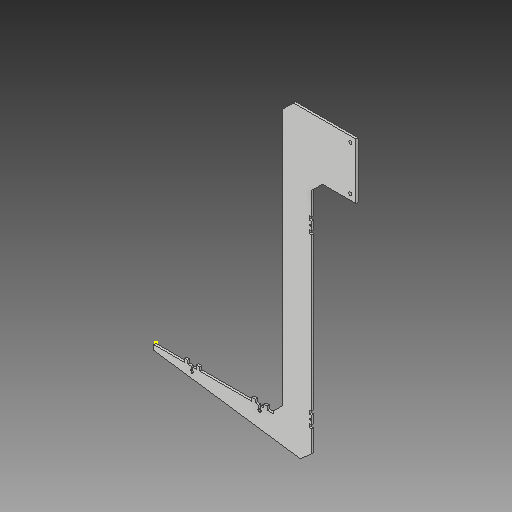
# Autodesk Inventor part: Z stage_side
Saved by Autodesk Inventor 2019 (Build 230136000, 136)
## iProperties
Created: 2020-03-07
Part Number: Z stage_side
Material: Generic
Document SubType Name: Modeling
Designer: Vijay
Density: 1 g/cm^3
Appearance: Default
Author: Vijay
Autodesk Inventor part; units mm, degrees
ref_plane "YZ Plane" through (0, 0, 0) normal (1, 0, 0) x (0, 1, 0)
ref_plane "XZ Plane" through (0, 0, 0) normal (0, 1, 0) x (-1, 0, 0)
ref_plane "XY Plane" through (0, 0, 0) normal (0, 0, 1) x (1, 0, 0)
sketch "Sketch1" plane through (0, 0, 0) normal (0, 0, 1) x (1, 0, 0)
  line L0 (230, 0) -> (0, 0) projected
  line L1 (0, 0) -> (0, -8.9243)
  line L2 (0, -8.9243) -> (282.1829, -48.5825)
  line L3 (282.1829, -48.5825) -> (282.1829, 400)
  line L4 (230, 0) -> (230, 500)
  line L5 (282.1829, 400) -> (362.1829, 400)
  line L6 (230, 500) -> (362.1829, 500)
  line L7 (362.1829, 500) -> (362.1829, 400)
  dimension "d0" = 400
  dimension "d1" = 8
  dimension "d10" = 80
  dimension "d11" = 100
  constraints: 14 end point, 2 horizontal, 2 vertical, 1 parallel, 1 perpendicular
  measures "d0" distance between parallel lines of L0 L5
  measures "d1" angle of L2 L0
  measures "d10" distance between parallel lines of L7 L3
  measures "d11" distance of L6.end L5.end
extrude "Extrusion1" add sketch "Sketch1" along normal blind 4
chamfer "Chamfer1" distance 20 angle 45 2 edges at (230, 500, 2) (282.1829, 400, 2)
chamfer "Chamfer2" distance 20 angle 45 2 edges at (230, 0, 2) (282.1829, -48.5825, 2)
sketch "Sketch2" plane through (0, 0, 0) normal (0, 0, -1) x (-1, 0, 0)
  point P0 (0, 0)
sketch "Sketch3" plane through (0, 0, 0) normal (0, 0, -1) x (-1, 0, 0)
  point P0 (0, 0)
sketch "Sketch4" plane through (0, 0, 0) normal (0, 0, -1) x (-1, 0, 0)
  point P0 (0, 0)
sketch "Sketch5" plane through (0, 0, 0) normal (0, 0, -1) x (-1, 0, 0)
  line L0 (-278.1829, 10.465) -> (-278.1829, 16.465) construction
  line L1 (-282.1829, 16.465) -> (-278.1829, 16.465) construction
  line L2 (-282.1829, 10.465) -> (-282.1829, 16.465) construction
  line L3 (-282.1829, 10.465) -> (-278.1829, 10.465) construction
  line L4 (-278.1829, 31.665) -> (-278.1829, 37.665) construction
  line L5 (-282.1829, 37.665) -> (-278.1829, 37.665) construction
  line L6 (-282.1829, 31.665) -> (-282.1829, 37.665) construction
  line L7 (-282.1829, 31.665) -> (-278.1829, 31.665) construction
  line L8 (-278.1829, 332.8339) -> (-278.1829, 338.8339) construction
  line L9 (-282.1829, 338.8339) -> (-278.1829, 338.8339) construction
  line L10 (-282.1829, 332.8339) -> (-282.1829, 338.8339) construction
  line L11 (-282.1829, 332.8339) -> (-278.1829, 332.8339) construction
  line L12 (-278.1829, 311.6339) -> (-278.1829, 317.6339) construction
  line L13 (-282.1829, 317.6339) -> (-278.1829, 317.6339) construction
  line L14 (-282.1829, 311.6339) -> (-282.1829, 317.6339) construction
  line L15 (-282.1829, 311.6339) -> (-278.1829, 311.6339) construction
  line L16 (-278.0829, 338.9339) -> (-278.0829, 332.7339)
  line L17 (-278.0829, 332.7339) -> (-282.2829, 332.7339)
  line L18 (-282.2829, 332.7339) -> (-282.2829, 338.9339)
  line L19 (-282.2829, 338.9339) -> (-278.0829, 338.9339)
  line L20 (-278.0829, 317.7339) -> (-278.0829, 311.5339)
  line L21 (-278.0829, 311.5339) -> (-282.2829, 311.5339)
  line L22 (-282.2829, 311.5339) -> (-282.2829, 317.7339)
  line L23 (-282.2829, 317.7339) -> (-278.0829, 317.7339)
  line L24 (-278.0829, 37.765) -> (-278.0829, 31.565)
  line L25 (-278.0829, 31.565) -> (-282.2829, 31.565)
  line L26 (-282.2829, 31.565) -> (-282.2829, 37.765)
  line L27 (-282.2829, 37.765) -> (-278.0829, 37.765)
  line L28 (-278.0829, 10.365) -> (-278.0829, 16.565)
  line L29 (-278.0829, 16.565) -> (-282.2829, 16.565)
  line L30 (-282.2829, 16.565) -> (-282.2829, 10.365)
  line L31 (-282.2829, 10.365) -> (-278.0829, 10.365)
  point P0 (0, 0)
  dimension "d24" = 0.1
  dimension "d25" = 0.1
  dimension "d26" = 0.1
  dimension "d27" = 0.1
  constraints: 32 end point, 12 other
  measures "d24" distance between parallel lines of L9 L19
  measures "d25" distance between parallel lines of L13 L23
  measures "d26" distance between parallel lines of L5 L27
  measures "d27" distance between parallel lines of L3 L31
extrude "Extrusion2" cut sketch "Sketch5" against normal blind 25.4
sketch "Sketch6" plane through (0, 0, 0) normal (0, 0, -1) x (-1, 0, 0)
  line L0 (-278.1829, 25.5649) -> (-278.1829, 22.5649) projected
  line L1 (-282.1829, 25.5649) -> (-278.1829, 25.5649) projected
  line L2 (-282.1829, 22.5649) -> (-282.1829, 25.5649) projected
  line L3 (-282.1829, 22.5649) -> (-278.1829, 22.5649) projected
  line L4 (-278.1829, 326.7338) -> (-278.1829, 323.7338) projected
  line L5 (-282.1829, 326.7338) -> (-278.1829, 326.7338) projected
  line L6 (-282.1829, 323.7338) -> (-282.1829, 326.7338) projected
  line L7 (-282.1829, 323.7338) -> (-278.1829, 323.7338) projected
  circle A0 centre (-280.1829, 325.2338) radius 1.5
  circle A1 centre (-280.1829, 24.0649) radius 1.5
  point P0 (0, 0)
  dimension "d14" = 3
  dimension "d15" = 3
  constraints: 2 centre point
  measures "d14" diameter of A0
  measures "d15" diameter of A1
extrude "Extrusion3" cut sketch "Sketch6" against normal through all contours A1 | A0
sketch "Sketch7" plane through (0, 0, 0) normal (0, 0, -1) x (-1, 0, 0)
  line L0 (-230, 4.0001) -> (-214.0001, 4.0001) projected
  line L1 (-210, 0) -> (-230, 20) projected
  line L2 (-210, 0) -> (-214.0001, 0)
  line L3 (-214.0001, 0) -> (-214.0001, 4.0001)
  line L4 (-214.0001, 4.0001) -> (-210, 4.0001)
  line L5 (-210, 4.0001) -> (-210, 0)
  point P0 (0, 0)
  constraints: 8 end point, 2 parallel, 2 point on line, 1 horizontal, 1 perpendicular
extrude "Extrusion4" cut sketch "Sketch7" against normal blind 25.4
sketch "Sketch8" plane through (0, 0, 0) normal (0, 0, -1) x (-1, 0, 0)
  line L0 (-209.8759, -14.6536) -> (-209.8759, 0) projected
  line L1 (-168.9242, -14.6536) -> (-209.8759, -14.6536) projected
  line L2 (-168.9242, 0) -> (-168.9242, -14.6536) projected
  line L3 (-175.8001, 0) -> (-168.9242, 0) projected
  line L4 (-175.8001, 6.35) -> (-175.8001, 0) projected
  line L5 (-181.8001, 6.35) -> (-175.8001, 6.35) projected
  line L6 (-181.8001, 0) -> (-181.8001, 6.35) projected
  line L7 (-187.9001, 0) -> (-181.8001, 0) projected
  line L8 (-187.9001, -6) -> (-187.9001, 0) projected
  line L9 (-186.6501, -6) -> (-187.9001, -6) projected
  line L10 (-186.6501, -8) -> (-186.6501, -6) projected
  line L11 (-187.9001, -8) -> (-186.6501, -8) projected
  line L12 (-187.9001, -10.65) -> (-187.9001, -8) projected
  line L13 (-190.9, -10.65) -> (-187.9001, -10.65) projected
  line L14 (-190.9, -8) -> (-190.9, -10.65) projected
  line L15 (-192.15, -8) -> (-190.9, -8) projected
  line L16 (-192.15, -6) -> (-192.15, -8) projected
  line L17 (-190.9, -6) -> (-192.15, -6) projected
  line L18 (-190.9, 0) -> (-190.9, -6) projected
  line L19 (-197, 0) -> (-190.9, 0) projected
  line L20 (-197, 6.35) -> (-197, 0) projected
  line L21 (-203.0001, 6.35) -> (-197, 6.35) projected
  line L22 (-203.0001, 0) -> (-203.0001, 6.35) projected
  line L23 (-209.8759, 0) -> (-203.0001, 0) projected
  line L24 (-88.9242, -14.6536) -> (-88.9242, 0) projected
  line L25 (-47.9725, -14.6536) -> (-88.9242, -14.6536) projected
  line L26 (-47.9725, 0) -> (-47.9725, -14.6536) projected
  line L27 (-54.8484, 0) -> (-47.9725, 0) projected
  line L28 (-54.8484, 6.35) -> (-54.8484, 0) projected
  line L29 (-60.8484, 6.35) -> (-54.8484, 6.35) projected
  line L30 (-60.8484, 0) -> (-60.8484, 6.35) projected
  line L31 (-66.9484, 0) -> (-60.8484, 0) projected
  line L32 (-66.9484, -6) -> (-66.9484, 0) projected
  line L33 (-65.6984, -6) -> (-66.9484, -6) projected
  line L34 (-65.6984, -8) -> (-65.6984, -6) projected
  line L35 (-66.9484, -8) -> (-65.6984, -8) projected
  line L36 (-66.9484, -10.65) -> (-66.9484, -8) projected
  line L37 (-69.9484, -10.65) -> (-66.9484, -10.65) projected
  line L38 (-69.9484, -8) -> (-69.9484, -10.65) projected
  line L39 (-71.1984, -8) -> (-69.9484, -8) projected
  line L40 (-71.1984, -6) -> (-71.1984, -8) projected
  line L41 (-69.9484, -6) -> (-71.1984, -6) projected
  line L42 (-69.9484, 0) -> (-69.9484, -6) projected
  line L43 (-76.0484, 0) -> (-69.9484, 0) projected
  line L44 (-76.0484, 6.35) -> (-76.0484, 0) projected
  line L45 (-82.0484, 6.35) -> (-76.0484, 6.35) projected
  line L46 (-82.0484, 0) -> (-82.0484, 6.35) projected
  line L47 (-88.9242, 0) -> (-82.0484, 0) projected
  point P0 (0, 0)
extrude "Extrusion5" add sketch "Sketch8" against normal up to surface (4 mm away)
sketch "Sketch10" plane through (0, 0, 0) normal (0, 0, -1) x (-1, 0, 0)
  line L0 (-209.8759, -14.6536) -> (-209.8759, 0) projected
  line L1 (-168.9242, -14.6536) -> (-209.8759, -14.6536) projected
  line L2 (-168.9242, 0) -> (-168.9242, -14.6536) projected
  line L3 (-175.8001, 0) -> (-168.9242, 0) projected
  line L4 (-175.8001, 6.35) -> (-175.8001, 0) projected
  line L5 (-181.8001, 6.35) -> (-175.8001, 6.35) projected
  line L6 (-181.8001, 0) -> (-181.8001, 6.35) projected
  line L7 (-187.9001, 0) -> (-181.8001, 0) projected
  line L8 (-187.9001, -6) -> (-187.9001, 0) projected
  line L9 (-186.6501, -6) -> (-187.9001, -6) projected
  line L10 (-186.6501, -8) -> (-186.6501, -6) projected
  line L11 (-187.9001, -8) -> (-186.6501, -8) projected
  line L12 (-187.9001, -10.65) -> (-187.9001, -8) projected
  line L13 (-190.9, -10.65) -> (-187.9001, -10.65) projected
  line L14 (-190.9, -8) -> (-190.9, -10.65) projected
  line L15 (-192.15, -8) -> (-190.9, -8) projected
  line L16 (-192.15, -6) -> (-192.15, -8) projected
  line L17 (-190.9, -6) -> (-192.15, -6) projected
  line L18 (-190.9, 0) -> (-190.9, -6) projected
  line L19 (-197, 0) -> (-190.9, 0) projected
  line L20 (-197, 6.35) -> (-197, 0) projected
  line L21 (-203.0001, 6.35) -> (-197, 6.35) projected
  line L22 (-203.0001, 0) -> (-203.0001, 6.35) projected
  line L23 (-209.8759, 0) -> (-203.0001, 0) projected
  line L24 (-88.9242, -14.6536) -> (-88.9242, 0) projected
  line L25 (-47.9725, -14.6536) -> (-88.9242, -14.6536) projected
  line L26 (-47.9725, 0) -> (-47.9725, -14.6536) projected
  line L27 (-54.8484, 0) -> (-47.9725, 0) projected
  line L28 (-54.8484, 6.35) -> (-54.8484, 0) projected
  line L29 (-60.8484, 6.35) -> (-54.8484, 6.35) projected
  line L30 (-60.8484, 0) -> (-60.8484, 6.35) projected
  line L31 (-66.9484, 0) -> (-60.8484, 0) projected
  line L32 (-66.9484, -6) -> (-66.9484, 0) projected
  line L33 (-65.6984, -6) -> (-66.9484, -6) projected
  line L34 (-65.6984, -8) -> (-65.6984, -6) projected
  line L35 (-66.9484, -8) -> (-65.6984, -8) projected
  line L36 (-66.9484, -10.65) -> (-66.9484, -8) projected
  line L37 (-69.9484, -10.65) -> (-66.9484, -10.65) projected
  line L38 (-69.9484, -8) -> (-69.9484, -10.65) projected
  line L39 (-71.1984, -8) -> (-69.9484, -8) projected
  line L40 (-71.1984, -6) -> (-71.1984, -8) projected
  line L41 (-69.9484, -6) -> (-71.1984, -6) projected
  line L42 (-69.9484, 0) -> (-69.9484, -6) projected
  line L43 (-76.0484, 0) -> (-69.9484, 0) projected
  line L44 (-76.0484, 6.35) -> (-76.0484, 0) projected
  line L45 (-82.0484, 6.35) -> (-76.0484, 6.35) projected
  line L46 (-82.0484, 0) -> (-82.0484, 6.35) projected
  line L47 (-88.9242, 0) -> (-82.0484, 0) projected
  line L48 (-190.9, 0) -> (-187.9001, 0)
  line L49 (-197, 0) -> (-181.8001, 0) projected
  line L50 (-69.9484, 0) -> (-66.9484, 0)
  line L51 (-76.0484, 0) -> (-60.8484, 0) projected
  point P0 (0, 0)
  constraints: 4 end point, 2 collinear
extrude "Extrusion6" cut sketch "Sketch10" against normal blind 25.4 contours L48 L8 L9 L10 L11 L12 L13 L14 L15 L16 L17 L18 | L50 L32 L33 L34 L35 L36 L37 L38 L39 L40 L41 L42
sketch "Sketch11" plane through (0, 0, 0) normal (0, 0, -1) x (-1, 0, 0)
  line L0 (-342.1829, 500) -> (-342.1829, 400) projected
  circle A0 centre (-352.1829, 490) radius 3
  circle A1 centre (-352.1829, 410) radius 3
  line L1 (-362.1829, 500) -> (-362.1829, 400) projected
  line L2 (-250, 500) -> (-362.1829, 500) projected
  line L3 (-362.1829, 400) -> (-302.1829, 400) projected
  point P0 (0, 0)
  dimension "d28" = 6
  dimension "d29" = 6
  dimension "d30" = 10
  dimension "d31" = 10
  dimension "d32" = 10
  dimension "d33" = 10
  constraints: 2 centre point
  measures "d28" diameter of A0
  measures "d29" diameter of A1
  measures "d30" distance from line of L1 A0.centre
  measures "d31" distance from line of L1 A1.centre
  measures "d32" distance from line of L2 A0.centre
  measures "d33" distance from line of L3 A1.centre
extrude "Extrusion7" cut sketch "Sketch11" against normal blind 25.4 contours A0 | A1
body "Solid1"
